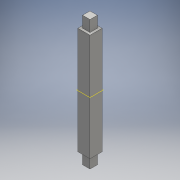
# Autodesk Inventor part: Upper Beam Support
Saved by Autodesk Inventor 2016 (Build 200138000, 138)
## iProperties
Created: 2016-03-08
Part Number: Upper Beam Support
Material: Generic
Document SubType Name: Modeling
Designer: Kenneth Daniel
Density: 1 g/cm^3
Appearance: Default
Mass: 32.725 g
Surface Area: 95.5 cm^2
Volume: 32.725 cm^3
Author: Kenneth Daniel
Autodesk Inventor part; units mm, degrees
ref_plane "YZ Plane" through (0, 0, 0) normal (1, 0, 0) x (0, 1, 0)
ref_plane "XZ Plane" through (0, 0, 0) normal (0, 1, 0) x (-1, 0, 0)
ref_plane "XY Plane" through (0, 0, 0) normal (0, 0, 1) x (1, 0, 0)
sketch "Sketch1" plane through (0, 0, 0) normal (0, 0, 1) x (1, 0, 0)
  line L0 (-7.5, -7.5) -> (7.5, -7.5)
  line L1 (7.5, -7.5) -> (7.5, 7.5)
  line L2 (7.5, 7.5) -> (-7.5, 7.5)
  line L3 (-7.5, 7.5) -> (-7.5, -7.5)
  line L4 (-7.5, -7.5) -> (7.5, 7.5) construction
  line L5 (7.5, -7.5) -> (-7.5, 7.5) construction
  point P0 (0, 0)
  dimension "d0" = 15
  dimension "d1" = 15
  constraints: 12 end point, 2 midpoint, 2 parallel, 1 horizontal, 1 perpendicular
  measures "d0" distance of L0.start L0.end
  measures "d1" distance of L1.end L0.end
extrude "Extrusion1" add sketch "Sketch1" along normal blind 133
ref_plane "Work Plane1" through (0, 0, 66.5) normal (0, 0, 1) x (1, 0, 0)
sketch "Sketch2" plane through (0, 0, 133) normal (0, 0, 1) x (1, 0, 0)
  line L0 (-5, -5) -> (5, -5)
  line L1 (5, -5) -> (5, 5)
  line L2 (5, 5) -> (-5, 5)
  line L3 (-5, 5) -> (-5, -5)
  line L4 (-5, -5) -> (5, 5) construction
  line L5 (5, -5) -> (-5, 5) construction
  point P0 (0, 0)
  dimension "d4" = 10
  dimension "d5" = 10
  constraints: 12 end point, 2 midpoint, 2 parallel, 1 horizontal, 1 perpendicular
  measures "d4" distance of L0.start L0.end
  measures "d5" distance of L1.end L0.end
extrude "Extrusion2" add sketch "Sketch2" along normal blind 14
mirror "Mirror1" about plane through (0, 0, 66.5) normal (0, 0, 1) of "Extrusion2"
sketch "Sketch3" plane through (0, 0, 147) normal (0, 0, 1) x (1, 0, 0)
  line L0 (-5, -5) -> (5, -5) projected
  line L1 (5, -5) -> (5, 5) projected
  line L2 (5, 5) -> (-5, 5) projected
  line L3 (-5, 5) -> (-5, -5) projected
  line L4 (-4.6, -4.6) -> (4.6, -4.6)
  line L5 (4.6, -4.6) -> (4.6, 4.6)
  line L6 (4.6, 4.6) -> (-4.6, 4.6)
  line L7 (-4.6, 4.6) -> (-4.6, -4.6)
  point P0 (0, 0)
  dimension "d8" = 0.4
  constraints: 8 end point, 3 other
  measures "d8" distance between parallel lines of L3 L7
extrude "Extrusion3" cut sketch "Sketch3" against normal up to surface (14 mm away)
mirror "Mirror2" about plane through (0, 0, 66.5) normal (0, 0, 1) of "Extrusion2"
mirror "Mirror3" about plane through (0, 0, 66.5) normal (0, 0, 1) of "Extrusion3"
body "Solid1"
